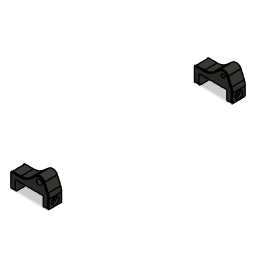
wheelstand base covers v4 (Autodesk Fusion 360 design; units mm, degrees)
Autodesk Fusion 360 part; units mm, degrees
sketch "Sketch1" plane through (0, 0, 0) normal (0, 0, 1) x (1, 0, 0)
  line L0 (-40.1, 0) -> (40.1, 0)
  line L1 (40.1, 0) -> (40.1, -30)
  line L2 (40.1, -30) -> (55.1, -30)
  line L3 (55.1, -30) -> (55.1, -2.1482)
  line L4 (52.2971, 11.5757) -> (42.6188, 34.2817)
  circle A0 centre (28.82, 28.4) radius 15
  circle A1 centre (28.82, 28.4) radius 4.5
  line L5 (-40.1, 0) -> (-40.1, -30)
  line L6 (-40.1, -30) -> (-55.1, -30)
  line L7 (-55.1, -30) -> (-55.1, 10)
  line L8 (-50.1, 15) -> (-25.7242, 15)
  line L9 (1.8038, 25.1201) -> (19.1042, 39.8282)
  arc A2 (-25.7242, 15) -> (1.8038, 25.1201) centre (-25.7242, 57.5) ccw
  arc A3 (-50.1, 15) -> (-55.1, 10) centre (-50.1, 10) ccw
  arc A4 (55.1, -2.1482) -> (52.2971, 11.5757) centre (20.1, -2.1482) ccw
  circle A5 centre (28.82, 28.4) radius 7.5
  point P0 (55.1, 5)
  point P1 (-55.1, 15)
  point P2 (-10.1, 15)
  dimension "d1" = 80.2
  dimension "d2" = 15
  dimension "d3" = 11.28
  dimension "d4" = 28.4
  dimension "d5" = 30
  dimension "d6" = 9
  dimension "d7" = 5
  dimension "d8" = 30
  dimension "d9" = 15
  dimension "d10" = 15
  dimension "d13" = 45
  dimension "d14" = 42.5
  dimension "d15" = 5
  dimension "d16" = 35
  dimension "d19" = 15
  constraint horizontal L0
  constraint midpoint origin L0
  constraint perpendicular L0 L1
  constraint perpendicular L1 L2
  constraint perpendicular L2 L3
  constraint tangent L4 A0
  constraint coincident L4.end A0
  constraint concentric A0 A1
  constraint perpendicular L0 L5
  constraint perpendicular L5 L6
  constraint perpendicular L6 L7
  constraint collinear L2 L6
  constraint perpendicular L7 L8
  constraint coincident A0 L9.end
  constraint tangent A0 L9
  constraint coincident P2 L9
  constraint coincident P2 L8
  constraint tangent L9 A2
  constraint tangent L8 A2
  constraint coincident P1 L8
  constraint coincident P1 L7
  constraint tangent L8 A3
  constraint tangent L7 A3
  constraint coincident P0 L4
  constraint coincident P0 L3
  constraint tangent L4 A4
  constraint tangent L3 A4
  constraint concentric A0 A5
  measures "d1" distance of L0.start L0.end
  measures "d2" distance of L1.end L2.end
  measures "d3" distance of L1 A0.centre
  measures "d4" distance of L0 A0.centre
  measures "d5" diameter of A0
  measures "d6" diameter of A1
  measures "d7" distance of L0 P0
  measures "d8" distance of L0.end L1.end
  measures "d9" distance of L0 P1
  measures "d10" distance of L5.end L6.end
  measures "d13" distance of P1 P2
  measures "d14" radius of A2
  measures "d15" radius of A3
  measures "d16" radius of A4
  measures "d19" diameter of A5
extrude "Extrude1" add sketch "Sketch1" along normal blind 40 contours L0 L1 L2 L3 L4 A0 L5 L6 L7 L8 L9 A2 A3 A4 | A0 | A5 makes body 1
extrude "Extrude2" cut sketch "Sketch1" along normal blind 20 contours A5 bodies 1
fillet "Fillet1" radius 3.5 4 edges at (47.6, -30, 40) (47.6, -30, 0) (-47.6, -30, 0) (-47.6, -30, 40) on bodies 1
chamfer "Chamfer1" distance 2 angle 45 18 edges at (-11.0596, 17.6102, 40) (-37.9121, 15, 40) (-53.6355, 13.5355, 40) (-55.1, -10, 40) (55.1, -16.0741, 40) (54.3921, 4.8554, 40) (47.4579, 22.9287, 40) (32.2636, 42.9994, 40) (10.454, 32.4741, 40) (47.4579, 22.9287, 0) (32.2636, 42.9994, 0) (10.454, 32.4741, 0) (-11.0596, 17.6102, 0) (-37.9121, 15, 0) (-53.6355, 13.5355, 0) (-55.1, -10, 0) (55.1, -16.0741, 0) (54.3921, 4.8554, 0) on bodies 1
chamfer "Chamfer1" distance 0.4 angle 45 1 faces at (33.2976, 27.9519, 26.6667) on bodies 1
sketch "Sketch2" plane through (-40.1, 0, 0) normal (1, 0, 0) x (0, 0, -1)
  line L0 (0, -26.5) -> (0, 0)
  line L1 (0, 0) -> (-40, 0)
  line L2 (-40, 0) -> (-40, -26.5)
  line L3 (-36.5, -30) -> (-3.5, -30)
  circle A0 centre (-20, -15) radius 10.5
  circle A1 centre (-20, -15) radius 4.25
  arc A2 (-40, -26.5) -> (-36.5, -30) centre (-36.5, -26.5) ccw
  arc A3 (-3.5, -30) -> (0, -26.5) centre (-3.5, -26.5) ccw
  line L4 (0, -26.5) -> (0, -30) construction
  line L5 (0, -30) -> (-3.5, -30) construction
  line L6 (0, -30) -> (-40, 0) construction
  dimension "d22" = 21
  dimension "d23" = 8.5
  constraint concentric A0 A1
  constraint coincident L0.start A3.end
  constraint tangent A3 L4
  constraint coincident L3.end A3.start
  constraint tangent A3 L5
  constraint coincident L1.end L2.start
  constraint midpoint A0.centre L6
  measures "d22" diameter of A0
  measures "d23" diameter of A1
extrude "Extrude3" cut sketch "Sketch2" along normal mid plane 280 contours A0 | A1 bodies 1
extrude "Extrude4" add sketch "Sketch2" against normal blind 8 contours A0 bodies 1
extrude "Extrude5" add sketch "Sketch2" along normal blind 8 from surface at 80.2 contours A0 bodies 1
ref_plane "WorkPlane1" through (0, 7.3702, 284.9) normal (0, 0, 1) x (1, 0, 0)
mirror "Mirror1" about plane through (0, 7.3702, 284.9) normal (0, 0, 1) of bodies 1 makes body 2
copy_body "Body->Comp1" bodies 1 removing the originals makes body 3 in component "wheelstand base cover RH"
copy_body "Body->Comp2" bodies 2 removing the originals makes body 4 in component "wheelstand base cover LH"
component "wheelstand base cover RH" placed x (1, 0, 0) y (0, 1, 0) z (0, 0, 1) at (0, 0, 0)
component "wheelstand base cover LH" placed x (1, 0, 0) y (0, 1, 0) z (0, 0, 1) at (0, 0, 0)
equation "d3 = 20 mm - 8.72 mm"
equation "d4 = 30 mm - 1.6 mm"
equation "d33 = ( 489.8 / 2 ) * 1 mm"
named bodies: "wheelstand base cover RH", "wheelstand base cover LH"
